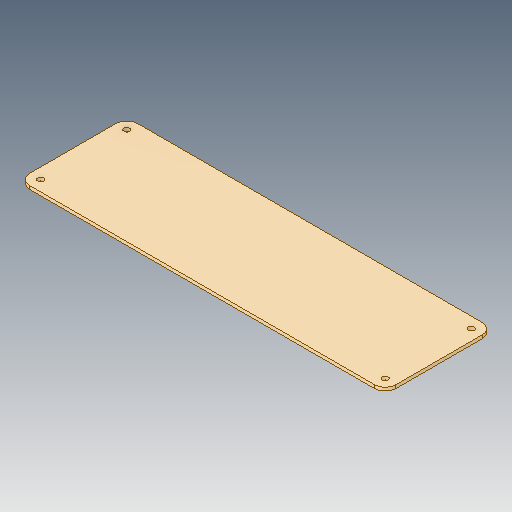
# Autodesk Inventor part: supportPlate
Saved by Autodesk Inventor 2018 (Build 220112000, 112)
## iProperties
Created: 2017-03-01
Part Number: supportPlate
Material: ABS Plastic
Document SubType Name: Modeling
Designer: sawaiz
Density: 1.06 g/cm^3
Appearance: Smooth - Off-White
Author: sawaiz
Autodesk Inventor part; units mm, degrees
ref_plane "YZ Plane" through (0, 0, 0) normal (1, 0, 0) x (0, 1, 0)
ref_plane "XZ Plane" through (0, 0, 0) normal (0, 1, 0) x (-1, 0, 0)
ref_plane "XY Plane" through (0, 0, 0) normal (0, 0, 1) x (1, 0, 0)
sketch "Sketch1" plane through (0, 0, 0) normal (0, 1, 0) x (-1, 0, 0)
  line L0 (170, 50) -> (-170, 50)
  line L1 (-170, 50) -> (-170, -50)
  line L2 (-170, -50) -> (170, -50)
  line L3 (170, -50) -> (170, 50)
  line L4 (170, 50) -> (-170, -50) construction
  line L5 (-170, 50) -> (170, -50) construction
  point P0 (0, 0)
  dimension "d0" = 340
  dimension "d1" = 100
  constraints: 12 end point, 2 midpoint, 2 parallel, 1 horizontal, 1 perpendicular
  measures "d0" distance of L2.end L1.end
  measures "d1" distance of L1.end L0.end
extrude "Extrusion1" add sketch "Sketch1" along normal mid plane 3.125
fillet "Fillet1" radius 10 4 edges at (-170, 0, 50) (-170, 0, -50) (170, 0, -50) (170, 0, 50)
sketch "Sketch2" plane through (0, 1.5625, 0) normal (0, 1, 0) x (1, 0, 0)
  arc A0 (160, -50) -> (170, -40) centre (160, -40) ccw projected
  line L0 (160, 50) -> (-160, 50) projected
  arc A1 (-160, 50) -> (-170, 40) centre (-160, 40) ccw projected
  line L1 (-160, -50) -> (160, -50) projected
  line L2 (170, -40) -> (170, 40) projected
  arc A2 (170, 40) -> (160, 50) centre (160, 40) ccw projected
  line L3 (-170, 40) -> (-170, -40) projected
  arc A3 (-170, -40) -> (-160, -50) centre (-160, -40) ccw projected
  point P0 (0, 0)
  dimension "d0" = 340
  dimension "d6" = 10
  dimension "d14" = 10
  measures "d6" distance from line of L1 point (-160, -40)
  measures "d14" distance from line of L3 point (-160, -40)
hole "Hole1" at (-160, 1.5625, 40) direction (0, -1, 0) diameter 5.5118 end through all clearance for "Socket Head Cap Screw" size "M5" standard "Ansi Metric M Profile"
mirror "Mirror1" about plane through (0, 0, 0) normal (0, 0, 1) of "Hole1"
mirror "Mirror2" about plane through (0, 0, 0) normal (1, 0, 0) of "Hole1", "Mirror1"
equation "\"d1\" = suppourtPlateLength"
equation "\"d2\" = acrylicThickness"
equation "\"suppourtPlateLength\" = 100"
equation "\"acrylicThickness\" = 3.125"
body "Solid1"
